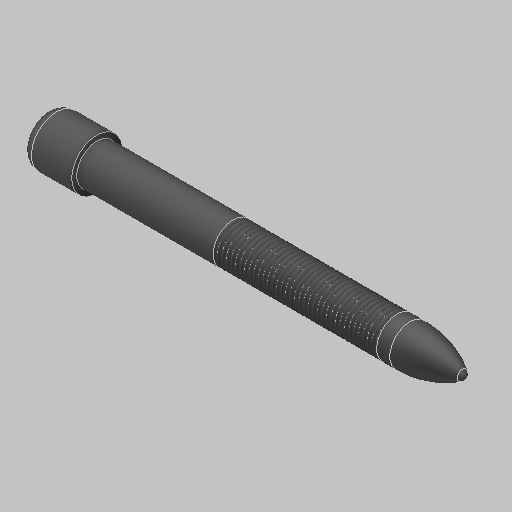
# Autodesk Inventor part: Caneta - IHM
Saved by Autodesk Inventor 2025.2 (Build 292293000, 293)
## iProperties
Created: 2024-09-25
Part Number: Caneta - IHM
Material: Genérico
Document SubType Name: Modeling
Designer: phmca
Density: 1 g/cm^3
Appearance: Padrão
Author: phmca
Autodesk Inventor part; units mm, degrees
ref_plane "YZ Plane" through (0, 0, 0) normal (1, 0, 0) x (0, 1, 0)
ref_plane "XZ Plane" through (0, 0, 0) normal (0, 1, 0) x (-1, 0, 0)
ref_plane "XY Plane" through (0, 0, 0) normal (0, 0, 1) x (1, 0, 0)
sketch "Esboço3" plane through (0, 0, 0) normal (0, 0, 1) x (1, 0, 0)
  arc A0 (37.45, 3.55) -> (37, 4) centre (37, 3.55) ccw
  line L0 (37, 3.55) -> (38.525, 3.55) construction
  arc A1 (38.35, 3.55) -> (37.45, 3.55) centre (37.9, 3.55) ccw
  line L1 (0, 0) -> (87.7294, 0) construction
  line L2 (0, 0) -> (0, 3)
  line L3 (2, 5) -> (10, 5)
  line L4 (10, 5) -> (10, 4)
  line L5 (10, 4) -> (37, 4)
  arc A2 (2, 5) -> (0, 3) centre (2, 3) ccw
  arc A3 (39.25, 3.55) -> (38.35, 3.55) centre (38.8, 3.55) ccw
  arc A4 (40.15, 3.55) -> (39.25, 3.55) centre (39.7, 3.55) ccw
  arc A5 (41.05, 3.55) -> (40.15, 3.55) centre (40.6, 3.55) ccw
  arc A6 (41.95, 3.55) -> (41.05, 3.55) centre (41.5, 3.55) ccw
  arc A7 (42.85, 3.55) -> (41.95, 3.55) centre (42.4, 3.55) ccw
  arc A8 (43.75, 3.55) -> (42.85, 3.55) centre (43.3, 3.55) ccw
  arc A9 (44.65, 3.55) -> (43.75, 3.55) centre (44.2, 3.55) ccw
  arc A10 (45.55, 3.55) -> (44.65, 3.55) centre (45.1, 3.55) ccw
  arc A11 (46.45, 3.55) -> (45.55, 3.55) centre (46, 3.55) ccw
  arc A12 (47.35, 3.55) -> (46.45, 3.55) centre (46.9, 3.55) ccw
  arc A13 (48.25, 3.55) -> (47.35, 3.55) centre (47.8, 3.55) ccw
  arc A14 (49.15, 3.55) -> (48.25, 3.55) centre (48.7, 3.55) ccw
  arc A15 (50.05, 3.55) -> (49.15, 3.55) centre (49.6, 3.55) ccw
  arc A16 (50.95, 3.55) -> (50.05, 3.55) centre (50.5, 3.55) ccw
  arc A17 (51.85, 3.55) -> (50.95, 3.55) centre (51.4, 3.55) ccw
  arc A18 (52.75, 3.55) -> (51.85, 3.55) centre (52.3, 3.55) ccw
  arc A19 (53.65, 3.55) -> (52.75, 3.55) centre (53.2, 3.55) ccw
  arc A20 (54.55, 3.55) -> (53.65, 3.55) centre (54.1, 3.55) ccw
  arc A21 (55.45, 3.55) -> (54.55, 3.55) centre (55, 3.55) ccw
  arc A22 (56.35, 3.55) -> (55.45, 3.55) centre (55.9, 3.55) ccw
  arc A23 (57.25, 3.55) -> (56.35, 3.55) centre (56.8, 3.55) ccw
  arc A24 (58.15, 3.55) -> (57.25, 3.55) centre (57.7, 3.55) ccw
  arc A25 (59.05, 3.55) -> (58.15, 3.55) centre (58.6, 3.55) ccw
  arc A26 (59.95, 3.55) -> (59.05, 3.55) centre (59.5, 3.55) ccw
  arc A27 (60.85, 3.55) -> (59.95, 3.55) centre (60.4, 3.55) ccw
  arc A28 (61.75, 3.55) -> (60.85, 3.55) centre (61.3, 3.55) ccw
  arc A29 (62.65, 3.55) -> (61.75, 3.55) centre (62.2, 3.55) ccw
  arc A30 (63.55, 3.55) -> (62.65, 3.55) centre (63.1, 3.55) ccw
  arc A31 (64.45, 3.55) -> (63.55, 3.55) centre (64, 3.55) ccw
  arc A32 (65.35, 3.55) -> (64.45, 3.55) centre (64.9, 3.55) ccw
  arc A33 (66.25, 3.55) -> (65.35, 3.55) centre (65.8, 3.55) ccw
  arc A34 (67.15, 3.55) -> (66.25, 3.55) centre (66.7, 3.55) ccw
  arc A35 (68.05, 3.55) -> (67.15, 3.55) centre (67.6, 3.55) ccw
  arc A36 (68.95, 3.55) -> (68.05, 3.55) centre (68.5, 3.55) ccw
  arc A37 (69.4, 4) -> (68.95, 3.55) centre (69.4, 3.55) ccw
  arc A38 (83, 0) -> (82.4032, 1.0658) centre (81.75, 0) ccw
  arc A39 (82.4032, 1.0658) -> (72, 4) centre (72, -15.9091) ccw
  line L6 (0, 0) -> (83, 0)
  line L7 (72, 4) -> (69.4, 4)
  line L8 (0, 0) -> (0.1769, 0) construction
  line L9 (0, 0) -> (0, 0.116) construction
  line L10 (37, 4) -> (69.4, 4) construction
  point P0 (37.45, 3.55)
  dimension "d8" = 0.9
  dimension "d9" = 0.9
  dimension "d10" = 1
  dimension "d11" = 2
  dimension "d14" = 0.9
  dimension "d19" = 0.9
  dimension "d20" = 2.5
  dimension "d21" = 5
  dimension "d22" = 10
  dimension "d23" = 4
  dimension "d25" = 72
  dimension "d26" = 83
  dimension "d29" = 0.45
  dimension "d31" = 32.4
  dimension "d32" = 37
  constraints: 81 point on circle, 40 centre point, 23 end point, 8 horizontal, 7 tangent, 3 collinear, 3 point on line, 2 vertical, 1 coincident, 136 other
  measures "d8" diameter of A0
  measures "d9" diameter of A1
  measures "d10" distance of L3.end L4.end
  measures "d11" radius of A2
  measures "d14" distance of A1.centre A3.centre
  measures "d19" diameter of A37
  measures "d20" diameter of A38
  measures "d21" distance between parallel lines of L3 L6
  measures "d22" distance between parallel lines of L4 L2
  measures "d23" distance between parallel lines of L6 L5
  measures "d25" distance from line of L2 L7.start
  measures "d26" distance of L1.start L6.end
  measures "d29" distance between parallel lines of L0 L5
  measures "d31" distance of L5.end A37.start
  measures "d32" distance from line of L2 L5.end
revolve "Revolução1" add sketch "Esboço3" angle 360 about axis through (0, 0, 0) along (1, 0, 0)
